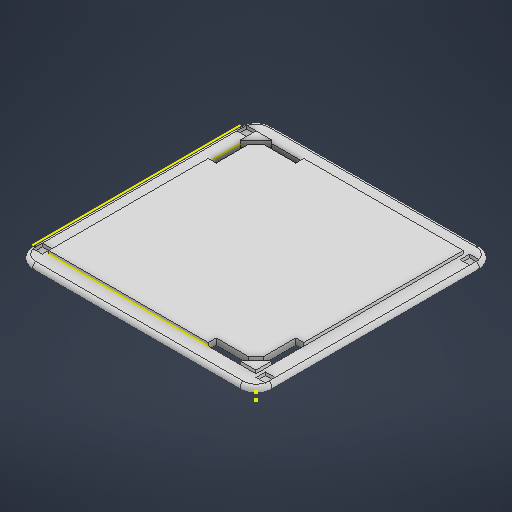
# Autodesk Inventor part: Tampa2.0
Saved by Autodesk Inventor 2026 (Build 300175050, 175E)
## iProperties
Created: 2025-03-23
Part Number: Tampa2.0
Material: Genérico
Document SubType Name: Modeling
Designer: miche
Density: 1 g/cm^3
Appearance: Padrão
Author: miche
Autodesk Inventor part; units mm, degrees
ref_plane "YZ Plane" through (0, 0, 0) normal (1, 0, 0) x (0, 1, 0)
ref_plane "XZ Plane" through (0, 0, 0) normal (0, 1, 0) x (-1, 0, 0)
ref_plane "XY Plane" through (0, 0, 0) normal (0, 0, 1) x (1, 0, 0)
sketch "Esboço1" plane through (0, 0, 0) normal (0, 1, 0) x (-1, 0, 0)
  line L0 (5, 0) -> (70, 0)
  line L1 (75, -5) -> (75, -70)
  line L2 (70, -75) -> (5, -75)
  line L3 (0, -70) -> (0, -5)
  arc A0 (70, -75) -> (75, -70) centre (70, -70) ccw
  arc A1 (0, -70) -> (5, -75) centre (5, -70) ccw
  arc A2 (75, -5) -> (70, 0) centre (70, -5) ccw
  arc A3 (5, 0) -> (0, -5) centre (5, -5) ccw
  point P0 (0, 0)
  point P1 (75, -75)
  point P2 (75, 0)
  point P3 (0, -75)
  dimension "d0" = 75
  dimension "d1" = 75
  dimension "d2" = 5
  constraints: 8 end point, 8 point on circle, 8 point on line, 8 tangent, 4 centre point, 3 equal radius, 2 parallel, 1 horizontal, 1 perpendicular
  measures "d0" distance of point (75, -75) point (0, -75)
  measures "d1" distance of point (75, 0) point (75, -75)
  measures "d2" radius of A0
extrude "Extrusão1" add sketch "Esboço1" along normal blind 3
sketch "Esboço3" plane through (0, 0, 0) normal (0, -1, 0) x (1, 0, 0)
  line L0 (-5, -75) -> (-70, -75) projected
  line L1 (-5, -75) -> (-5, -70)
  line L2 (-5, -70) -> (-70, -70)
  line L3 (-70, -70) -> (-70, -5)
  line L4 (-70, -5) -> (-5, -5)
  line L5 (-5, -5) -> (-5, -70)
  point P0 (0, 0)
  dimension "d14" = 5
  dimension "d15" = 65
  dimension "d16" = 65
  constraints: 10 end point, 2 parallel, 1 horizontal, 1 perpendicular, 1 vertical
  measures "d14" distance of L0.start L1.end
  measures "d15" distance of L3.end L4.end
  measures "d16" distance of L2.end L3.end
extrude "Extrusão3" cut sketch "Esboço3" against normal blind 1
sketch "Esboço4" plane through (0, 3, 0) normal (0, 1, 0) x (1, 0, 0)
  line L0 (-5, 70) -> (-70, 70) projected
  line L1 (-70, 70) -> (-65, 70)
  line L2 (-70, 70) -> (-70, 65)
  line L3 (-70, 65) -> (-65, 70)
  line L4 (-70, 5) -> (-5, 5) projected
  line L5 (-5, 5) -> (-5, 10)
  line L6 (-5, 5) -> (-5, 70) projected
  line L7 (-5, 5) -> (-10, 5)
  line L8 (-10, 5) -> (-5, 10)
  line L9 (-70, 65) -> (-70, 55)
  line L10 (-70, 70) -> (-70, 5) projected
  line L11 (-70, 55) -> (-67.5, 55)
  line L12 (-65, 70) -> (-55, 70)
  line L13 (-55, 70) -> (-55, 67.5)
  line L14 (-55, 67.5) -> (-63.9645, 67.5)
  line L15 (-65, 70) -> (-55, 70)
  line L16 (-70, 65) -> (-70, 55)
  line L17 (-67.5, 65) -> (-65, 67.5)
  line L18 (-67.5, 65) -> (-67.5, 55)
  line L19 (-65, 67.5) -> (-63.9645, 67.5)
  point P0 (0, 0)
  constraints: 32 end point, 5 point on line, 3 vertical, 2 horizontal, 2 perpendicular, 1 collinear
sketch "Esboço5" plane through (0, 3, 0) normal (0, 1, 0) x (1, 0, 0)
  line L0 (-5, 5) -> (-5, 70) projected
  line L1 (-5, 10) -> (-5, 20)
  line L2 (-5, 20) -> (-7.5, 20)
  line L3 (-70, 5) -> (-5, 5) projected
  line L4 (-10, 5) -> (-20, 5)
  line L5 (-20, 5) -> (-20, 7.5)
  line L6 (-7.5, 10) -> (-10, 7.5)
  line L7 (-7.5, 20) -> (-7.5, 10)
  line L8 (-20, 7.5) -> (-10, 7.5)
  line L9 (-5, 20) -> (-5, 10)
  line L10 (-20, 5) -> (-10, 5)
  line L11 (-10, 5) -> (-5, 10)
  point P0 (0, 0)
  dimension "d23" = 2.5
  dimension "d24" = 10
  dimension "d25" = 2.5
  constraints: 20 end point, 4 point on line, 3 perpendicular, 1 collinear, 1 vertical
  measures "d23" distance of L1.end L2.end
  measures "d24" distance of L4.start L4.end
  measures "d25" distance of L4.end L5.end
extrude "Extrusão4" cut sketch "Esboço5" against normal through all contours L11 L3 L5 L8 L6 L7 L2 L0
extrude "Extrusão5" cut sketch "Esboço4" against normal through all contours L13 L14 L19 L17 L18 L11 L9 L3 L0
sketch "Esboço6" plane through (0, 3, 0) normal (0, 1, 0) x (1, 0, 0)
  line L0 (-70, 70) -> (-70, 5) projected
  line L1 (-5, 5) -> (-5, 70) projected
  line L2 (-70, 70) -> (-5, 70)
  line L3 (-5, 70) -> (-5, 5)
  line L4 (-5, 5) -> (-70, 5)
  line L5 (-70, 5) -> (-70, 70)
  arc A0 (0, 70) -> (-5, 75) centre (-5, 70) ccw projected
  line L6 (-5, 75) -> (0, 75)
  line L7 (0, 75) -> (0, 0)
  line L8 (0, 0) -> (-5, 0)
  line L9 (-5, 0) -> (-5, 75)
  line L10 (-75, 75) -> (0, 75)
  line L11 (0, 75) -> (0, 70)
  line L12 (0, 70) -> (-75, 70)
  line L13 (-75, 70) -> (-75, 75)
  line L14 (0, 0) -> (-75, 0)
  line L15 (-75, 0) -> (-75, 5)
  line L16 (-75, 5) -> (0, 5)
  line L17 (0, 5) -> (0, 0)
  line L18 (-75, 0) -> (-70, 0)
  line L19 (-70, 0) -> (-70, 75)
  line L20 (-70, 75) -> (-75, 75)
  line L21 (-75, 75) -> (-75, 0)
  constraints: 40 end point, 10 parallel, 6 point on line, 5 horizontal, 5 perpendicular
extrude "Extrusão6" cut sketch "Esboço6" against normal blind 1 contours L19 L10 L9 L2 | L0 L16 L21 L12 | L12 L13 L10 L19 | L19 L14 L15 L16 | L4 L9 L14 L19 | L12 L7 L16 L1 | L9 A0 L12 | L16 L7 L8 L9 | L6 L7 A0
sketch "Esboço7" plane through (0, 0, -5) normal (1, 0, 0) x (0, 0, -1)
  point P0 (-5, 0)
sketch "Esboço8" plane through (0, 2, 0) normal (0, 1, 0) x (1, 0, 0)
  line L0 (-70, 5) -> (-20, 5) projected
  line L1 (-70, 5) -> (-70, 6.5)
  line L2 (-70, 70) -> (-70, 5) projected
  line L3 (-75, 70) -> (-75, 5) projected
  point P0 (0, 0)
  constraints: 2 end point, 1 point on line
fillet "Arredondamento1" radius 1 16 edges at (-73.5355, 2, -1.4645) (-75, 2, -37.5) (-73.5355, 2, -73.5355) (-37.5, 2, -75) (-1.4645, 2, -73.5355) (0, 2, -37.5) (-1.4645, 2, -1.4645) (-37.5, 2, 0) (-1.4645, 0, -1.4645) (0, 0, -37.5) (-1.4645, 0, -73.5355) (-37.5, 0, -75) (-73.5355, 0, -73.5355) (-75, 0, -37.5) (-73.5355, 0, -1.4645) (-37.5, 0, 0)
sketch "Esboço9" plane through (0, 2, 0) normal (0, 1, 0) x (1, 0, 0)
  line L0 (-70, 1) -> (-70, 0) projected
  line L1 (-70, 0) -> (-70, 4)
  line L2 (-74, 5) -> (-75, 5) projected
  line L3 (-75, 5) -> (-71, 5)
  line L4 (-70, 4) -> (-71, 4)
  line L5 (-71, 4) -> (-71, 5)
  line L6 (-74, 5) -> (-74, 70) projected
  line L7 (-71, 4) -> (-74, 4)
  line L8 (-74, 4) -> (-74, 7)
  line L9 (-74, 7) -> (-71, 7)
  line L10 (-71, 7) -> (-71, 4)
  line L11 (-5, 0) -> (-5, 1) projected
  line L12 (-5, 0) -> (-5, 4)
  line L13 (0, 4) -> (-4, 4)
  line L14 (-70, 74) -> (-70, 75) projected
  line L15 (-70, 75) -> (-70, 71)
  line L16 (-74, 70) -> (-75, 70) projected
  line L17 (-75, 70) -> (-71, 70)
  line L18 (-5, 74) -> (-5, 75) projected
  line L19 (-5, 75) -> (-5, 71)
  line L20 (0, 70) -> (-1, 70) projected
  line L21 (0, 70) -> (-4, 70)
  line L22 (-1, 70) -> (-1, 5) projected
  line L23 (-4, 71) -> (-1, 71)
  line L24 (-1, 71) -> (-1, 68)
  line L25 (-1, 68) -> (-4, 68)
  line L26 (-4, 68) -> (-4, 71)
  line L27 (-71, 71) -> (-74, 71)
  line L28 (-74, 71) -> (-74, 68)
  line L29 (-74, 68) -> (-71, 68)
  line L30 (-71, 68) -> (-71, 71)
  line L31 (-4, 4) -> (-1, 4)
  line L32 (-1, 4) -> (-1, 7)
  line L33 (-1, 7) -> (-4, 7)
  line L34 (-4, 7) -> (-4, 4)
  point P0 (0, 0)
  dimension "d43" = 4
  dimension "d44" = 4
  dimension "d45" = 3
  dimension "d46" = 4
  dimension "d47" = 4
  dimension "d50" = 4
  dimension "d51" = 4
  dimension "d52" = 4
  dimension "d53" = 4
  dimension "d54" = 3
  dimension "d55" = 3
  dimension "d56" = 3
  constraints: 52 end point, 9 horizontal, 8 parallel, 5 perpendicular, 5 point on line, 4 vertical
  measures "d43" distance of L0.end L1.end
  measures "d44" distance of L2.end L3.end
  measures "d45" distance of L7.end L8.end
  measures "d46" distance of L11.start L12.end
  measures "d47" distance of L13.start L13.end
  measures "d50" distance of L14.end L15.end
  measures "d51" distance of L16.end L17.end
  measures "d52" distance of L18.end L19.end
  measures "d53" distance of L20.start L21.end
  measures "d54" distance of L23.end L24.end
  measures "d55" distance of L33.end L32.end
  measures "d56" distance of L32.end L31.end
extrude "Extrusão7" cut sketch "Esboço9" against normal blind 1
